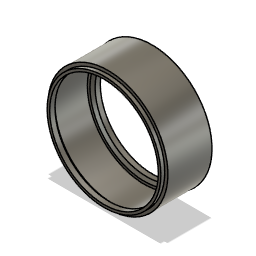
chamber body (Autodesk Fusion 360 design; units mm, degrees)
Autodesk Fusion 360 part; units mm, degrees
sketch "chamber" plane through (0, 0, 0) normal (0, 0, 1) x (1, 0, 0)
  circle A0 centre (0, 0) radius 43.825
  circle A1 centre (0, 0) radius 41.875
  circle A2 centre (0, 0) radius 46.25
  circle A3 centre (0, 0) radius 39.85
  dimension "d4" = 87.65
  dimension "d5" = 83.75
  dimension "d6" = 92.5
  dimension "d14" = 79.7
  constraint coincident A0.centre A1.centre
  constraint concentric A0 A3
  measures "d4" diameter of A0
  measures "d5" diameter of A1
  measures "d6" diameter of A2
  measures "d14" diameter of A3
extrude "Extrude1" add sketch "chamber" along normal blind 34 contours A2
extrude "Extrude3" add sketch "chamber" along normal blind 6 from surface at 31 contours A0
extrude "Extrude4" add sketch "chamber" along normal blind 6 contours A0 | A1
extrude "Extrude5" cut sketch "chamber" along normal blind 4 contours A0
chamfer "Chamfer1" distance 2 angle 45 1 edges at (-37.1532, 14.4104, 6)
chamfer "Chamfer2" distance 1.9 angle 45 1 edges at (-39.0412, 15.1426, 31)
equation "ChamberSize = 92.5 mm"
equation "ChamberOffset = 4.8 mm"
equation "ChamberInner = 4 mm"
equation "d4 = ChamberSize - ChamberOffset - 0.05 mm"
equation "d5 = ChamberSize - ChamberOffset - ChamberInner + 0.05 mm"
equation "d6 = ChamberSize"
equation "ChamberHeight = 34 mm"
equation "d8 = ChamberHeight"
equation "ChamberLip = 4 mm"
equation "d14 = ChamberSize - ChamberOffset - ChamberInner - 4 mm"
equation "d15 = ChamberLip + 2 mm"
equation "d17 = ChamberHeight - 3 mm"
named bodies: "chamber body"
